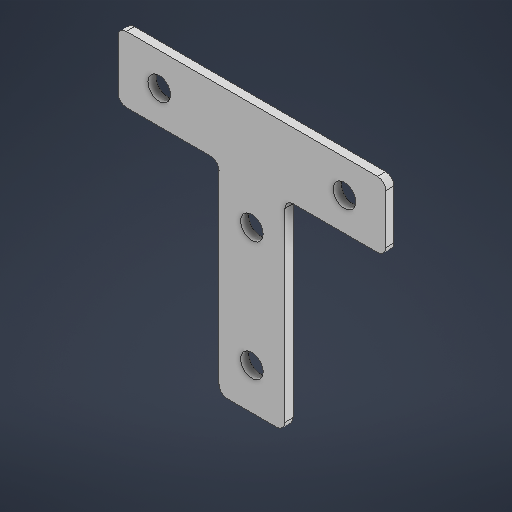
# Autodesk Inventor part: T型
Saved by Autodesk Inventor 2025 (Build 290162000, 162)
## iProperties
Created: 2025-06-23
Part Number: T型
Material: 常规
Document SubType Name: Modeling
Designer: HZD
Density: 1 g/cm^3
Appearance: 默认
Author: HZD
Autodesk Inventor part; units mm, degrees
ref_plane "YZ Plane" through (0, 0, 0) normal (1, 0, 0) x (0, 1, 0)
ref_plane "XZ Plane" through (0, 0, 0) normal (0, 1, 0) x (-1, 0, 0)
ref_plane "XY Plane" through (0, 0, 0) normal (0, 0, 1) x (1, 0, 0)
sketch "草图1" plane through (0, 0, 0) normal (0, 0, 1) x (1, 0, 0)
  line L0 (32.5, -8) -> (-32.5, -8)
  line L1 (-32.5, -8) -> (-32.5, 8)
  line L2 (-32.5, 8) -> (32.5, 8)
  line L3 (32.5, 8) -> (32.5, -8)
  line L4 (32.5, -8) -> (-32.5, 8) construction
  line L5 (-32.5, -8) -> (32.5, 8) construction
  line L6 (8, -57) -> (-8, -57)
  line L7 (-8, -57) -> (-8, 8)
  line L8 (-8, 8) -> (8, 8)
  line L9 (8, 8) -> (8, -57)
  line L10 (8, -57) -> (-8, 8) construction
  line L11 (-8, -57) -> (8, 8) construction
  line L12 (0, 0) -> (0, -24.5)
  point P0 (-8, -8)
  point P1 (8, -8)
  dimension "d0" = 65
  dimension "d1" = 16
  dimension "d2" = 49
  dimension "d3" = 16
  constraints: 26 end point, 4 midpoint, 4 parallel, 2 horizontal, 2 perpendicular, 1 point on line, 1 vertical
  measures "d0" distance of L1.end L2.end
  measures "d1" distance of L0.end L1.end
  measures "d2" distance between parallel lines of L6 L0
  measures "d3" distance of L6.start L6.end
extrude "拉伸1" add sketch "草图1" along normal blind 2
sketch "草图2" plane through (0, 0, 2) normal (0, 0, 1) x (1, 0, 0)
  line L0 (-32.5, 8) -> (-32.5, -8) projected
  line L1 (-32.5, 0) -> (32.5, 0)
  line L2 (32.5, -8) -> (32.5, 8) projected
  line L3 (0, 8) -> (0, -57)
  line L4 (-8, -57) -> (8, -57) projected
  circle A0 centre (-22.5, 0) radius 2.75
  circle A1 centre (0, -18) radius 2.75
  circle A2 centre (0, -47) radius 2.75
  circle A3 centre (22.5, 0) radius 2.75
  point P0 (0, 0)
  dimension "d6" = 22.5
  dimension "d7" = 5.5
  dimension "d8" = 5.5
  dimension "d9" = 5.5
  dimension "d10" = 29
  dimension "d11" = 10
  constraints: 4 centre point, 4 end point, 3 midpoint, 3 point on line, 1 symmetric about line, 1 vertical, 1 other
  measures "d6" distance from line of A0.centre L3
  measures "d7" diameter of A0
  measures "d8" diameter of A1
  measures "d9" diameter of A2
  measures "d10" distance of A2.centre A1.centre
  measures "d11" distance from line of A2.centre L4
extrude "拉伸2" cut sketch "草图2" against normal blind 10
fillet "圆角1" radius 2 8 edges at (-8, -8, 1) (-32.5, -8, 1) (-32.5, 8, 1) (32.5, -8, 1) (-8, -57, 1) (8, -57, 1) (8, -8, 1) (32.5, 8, 1)
equation "\"d12\" = d11"
